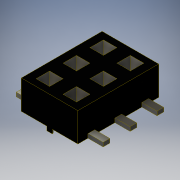
# Autodesk Inventor part: conn_2x3_2mm_FemaleSMT_M22-2540305
Saved by Autodesk Inventor 2016 (Build 200138000, 138)
## iProperties
Created: 2016-09-12
Part Number: conn_2x3_2mm_FemaleSMT_M22-2540305
Material: Generic
Document SubType Name: Modeling
Designer: jfixelle
Density: 1 g/cm^3
Appearance: Silver
Author: jfixelle
Autodesk Inventor part; units mm, degrees
ref_plane "YZ Plane" through (0, 0, 0) normal (1, 0, 0) x (0, 1, 0)
ref_plane "XZ Plane" through (0, 0, 0) normal (0, 1, 0) x (-1, 0, 0)
ref_plane "XY Plane" through (0, 0, 0) normal (0, 0, 1) x (1, 0, 0)
sketch "Sketch1" plane through (0, 0, 0) normal (0, 1, 0) x (-1, 0, 0)
  line L0 (2.1, 3) -> (-2.1, 3)
  line L1 (-2.1, 3) -> (-2.1, -3)
  line L2 (-2.1, -3) -> (2.1, -3)
  line L3 (2.1, -3) -> (2.1, 3)
  point P0 (0, 0)
  dimension "d0" = 6
  dimension "d1" = 3
  dimension "d2" = 4.2
  dimension "d3" = 2.1
  constraints: 8 end point, 2 parallel, 1 horizontal, 1 perpendicular
  measures "d0" distance of L2.end L0.start
  measures "d1" distance from line of L2 point (0, 0)
  measures "d2" distance of L1.end L2.end
  measures "d3" distance from line of point (0, 0) L3
extrude "Extrusion1" add sketch "Sketch1" along normal blind 2.15
sketch "Sketch2" plane through (0, 2.15, 0) normal (0, 1, 0) x (1, 0, 0)
  line L0 (-1.5, -0.5) -> (-0.5, -0.5)
  line L1 (-0.5, -0.5) -> (-0.5, 0.5)
  line L2 (-0.5, 0.5) -> (-1.5, 0.5)
  line L3 (-1.5, 0.5) -> (-1.5, -0.5)
  line L4 (-2.1, 3) -> (-2.1, -3) projected
  line L5 (-2.1, -2.6091) -> (-2.1, -0.2584)
  line L6 (-1.225, 3) -> (-0.0513, 3)
  line L7 (2.1, 3) -> (-2.1, 3) projected
  point P0 (0, 0)
  dimension "d6" = 1
  dimension "d7" = 1
  dimension "d8" = 0.5
  dimension "d9" = 0.5
  constraints: 12 end point, 3 point on line, 2 parallel, 1 horizontal, 1 perpendicular
  measures "d6" distance of L1.end L2.end
  measures "d7" distance of L0.end L1.end
  measures "d8" distance from line of point (0, 0) L1
  measures "d9" distance from line of point (0, 0) L2
extrude "Extrusion2" cut sketch "Sketch2" against normal through all
pattern_linear "Rectangular Pattern1" count 3 spacing 2 along (0, 0, 1) count 2 spacing 2 along (1, 0, 0) of "Extrusion2" first direction both ways yes
sketch "Sketch3" plane through (0, 0, 0) normal (0, -1, 0) x (1, 0, 0)
  line L0 (1.5, 0.5) -> (1.5, -0.5) projected
  line L1 (1.5, -0.25) -> (3.225, -0.25)
  line L2 (3.225, -0.25) -> (3.225, 0.25)
  line L3 (3.225, 0.25) -> (1.5, 0.25)
  line L4 (1.5, 0.25) -> (1.5, -0.25)
  line L5 (0.5, 0.5) -> (1.5, 0.5) projected
  point P0 (0, 0)
  dimension "d18" = 0.5
  dimension "d19" = 0.25
  dimension "d20" = 3.225
  constraints: 8 end point, 2 parallel, 1 horizontal, 1 perpendicular, 1 point on line
  measures "d18" distance of L1.end L2.end
  measures "d19" distance between parallel lines of L5 L3
  measures "d20" distance from line of point (0, 0) L2
extrude "Extrusion3" add sketch "Sketch3" against normal blind 0.3
pattern_linear "Rectangular Pattern2" count 3 spacing 2 along (0, 0, 1) of "Extrusion3" first direction both ways yes
mirror "Mirror1" about plane through (0, 0, 0) normal (1, 0, 0) of "Extrusion3", "Rectangular Pattern2"
sketch "Sketch4" plane through (0, 0, 0) normal (0, -1, 0) x (1, 0, 0)
  line L0 (-2.1, 3) -> (2.1, 3) projected
  arc A0 (-0.2, 3) -> (0.2, 3) centre (0, 3) ccw
  line L1 (2.1, -3) -> (-2.1, -3) projected
  arc A1 (0.2, -3) -> (-0.2, -3) centre (0, -3) ccw
  line L2 (0.2, 3) -> (-0.2, 3)
  line L3 (0.4327, -3) -> (-0.5599, -3)
  point P0 (0, 0)
  dimension "d26" = 0.4
  dimension "d27" = 0.4
  constraints: 5 point on line, 4 end point, 4 point on circle, 2 centre point, 2 midpoint
  measures "d26" diameter of A1
  measures "d27" diameter of A0
extrude "Extrusion4" add sketch "Sketch4" along normal blind 0.3
body "Solid1"
